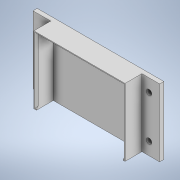
# Autodesk Inventor part: MediumHolder
Saved by Autodesk Inventor 2020 (Build 240168000, 168)
## iProperties
Created: 2023-03-07
Part Number: MediumHolder
Material: Generic
Document SubType Name: Modeling
Designer: DSOB
Density: 1 g/cm^3
Appearance: Default
Author: DSOB
Autodesk Inventor part; units mm, degrees
ref_plane "YZ Plane" through (0, 0, 0) normal (1, 0, 0) x (0, 1, 0)
ref_plane "XZ Plane" through (0, 0, 0) normal (0, 1, 0) x (-1, 0, 0)
ref_plane "XY Plane" through (0, 0, 0) normal (0, 0, 1) x (1, 0, 0)
sketch "Sketch1" plane through (0, 0, 0) normal (0, 0, 1) x (1, 0, 0)
  line L0 (0, 0) -> (150, 0)
  line L1 (150, 0) -> (150, 80)
  line L2 (150, 80) -> (0, 80)
  line L3 (0, 80) -> (0, 0)
  dimension "d0" = 150
  dimension "d1" = 80
  constraints: 8 end point, 2 parallel, 1 horizontal, 1 perpendicular
  measures "d0" distance of L1.end L2.end
  measures "d1" distance of L0.end L1.end
extrude "Extrusion1" add sketch "Sketch1" along normal blind 5
sketch "Sketch2" plane through (0, 0, 5) normal (0, 0, 1) x (1, 0, 0)
  line L0 (0, 0) -> (150, 0) projected
  line L1 (150, 80) -> (0, 80) projected
  line L2 (129, 0) -> (21, 0)
  line L3 (21, 0) -> (21, 80)
  line L4 (21, 80) -> (129, 80)
  line L5 (129, 80) -> (129, 0)
  line L6 (126, 3) -> (24, 3)
  line L7 (24, 3) -> (24, 77)
  line L8 (24, 77) -> (126, 77)
  line L9 (126, 77) -> (126, 3)
  line L10 (150, 0) -> (150, 80) projected
  point P0 (129, 80)
  point P1 (21, 0)
  dimension "d4" = 108
  dimension "d5" = 102
  dimension "d6" = 3
  dimension "d7" = 3
  dimension "d8" = 3
  dimension "d9" = 21
  constraints: 16 end point, 4 parallel, 2 horizontal, 2 perpendicular, 2 point on line
  measures "d4" distance between parallel lines of L3 L5
  measures "d5" distance of L6.start L6.end
  measures "d6" distance between parallel lines of L3 L7
  measures "d7" distance between parallel lines of L0 L6
  measures "d8" distance between parallel lines of L1 L8
  measures "d9" distance between parallel lines of L5 L10
extrude "Extrusion2" add sketch "Sketch2" along normal blind 20 contours L3 L1 L5 L0
chamfer "Chamfer1" distance 2 angle 45 1 edges at (75, 3, 25)
chamfer "Chamfer2" distance 2 angle 45 1 edges at (126, 40, 25)
chamfer "Chamfer3" distance 2 angle 45 2 edges at (75, 77, 25) (24, 40, 25)
sketch "Sketch3" plane through (0, 0, 5) normal (0, 0, 1) x (1, 0, 0)
  circle A0 centre (137.5, 15) radius 3.25
  circle A1 centre (137.5, 65) radius 3.25
  line L0 (150, 0) -> (150, 80) projected
  line L1 (129, 0) -> (150, 0) projected
  line L2 (75, -16.6248) -> (75, 70.7208)
  line L3 (0, 80) -> (0, 0) projected
  circle A2 centre (12.5, 15) radius 3.25
  circle A3 centre (12.5, 65) radius 3.25
  dimension "d21" = 6.5
  dimension "d22" = 6.5
  dimension "d23" = 12.5
  dimension "d24" = 12.5
  dimension "d25" = 50
  dimension "d26" = 15
  dimension "d27" = 75
  constraints: 4 centre point, 2 end point, 2 symmetric about line, 1 vertical, 2 other
  measures "d21" diameter of A0
  measures "d22" diameter of A1
  measures "d23" distance from line of L0 A0.centre
  measures "d24" distance from line of L0 A1.centre
  measures "d25" distance of A0.centre A1.centre
  measures "d26" distance from line of L1 A0.centre
  measures "d27" distance between parallel lines of L3 L2
extrude "Extrusion3" cut sketch "Sketch3" against normal blind 60
sketch "Sketch4" plane through (24, 3, 5) normal (0, 1, 0) x (1, 0, 0)
  line L0 (0, 0) -> (0, -18) projected
  line L1 (102, -18) -> (102, 10.1304)
  line L2 (102, 10.1304) -> (0, 10.1304)
  line L3 (0, 10.1304) -> (0, -18)
  line L4 (0, 0) -> (102, 0) projected
  line L5 (102, 0) -> (0, 0)
  line L6 (0, 0) -> (0, -34.2808)
  line L7 (0, -34.2808) -> (102, -34.2808)
  line L8 (102, -34.2808) -> (102, 0)
  point P0 (-24, 5)
  constraints: 14 end point, 3 parallel, 1 horizontal, 1 perpendicular
extrude "Extrusion5" cut sketch "Sketch4" against normal blind 10 contours L4 L1 L8 L7 L6 L0
fillet "Fillet1" radius 2 1 edges at (127, 1, 25)
fillet "Fillet2" radius 1 3 edges at (126, 0.9369, 24.8478) (126, 0.0858, 25) (126, 2.2929, 23.7071)
body "Solid1"
